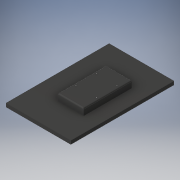
# Autodesk Inventor part: SpectreE165W_16in
Saved by Autodesk Inventor 2019 (Build 230136000, 136)
## iProperties
Created: 2019-05-22
Part Number: SpectreE165W_16in
Material: Generic
Document SubType Name: Modeling
Designer: Jorian Bruslind
Density: 1 g/cm^3
Appearance: Default
Author: Jorian Bruslind
Autodesk Inventor part; units mm, degrees
ref_plane "YZ Plane" through (0, 0, 0) normal (1, 0, 0) x (0, 1, 0)
ref_plane "XZ Plane" through (0, 0, 0) normal (0, 1, 0) x (-1, 0, 0)
ref_plane "XY Plane" through (0, 0, 0) normal (0, 0, 1) x (1, 0, 0)
sketch "Sketch1" plane through (0, 0, 0) normal (0, 1, 0) x (-1, 0, 0)
  line L0 (0, 0) -> (236.22, 0)
  line L1 (236.22, 0) -> (236.22, -375.92)
  line L2 (236.22, -375.92) -> (0, -375.92)
  line L3 (0, -375.92) -> (0, 0)
  dimension "d0" = 236.22
  dimension "d1" = 375.92
  constraints: 8 end point, 2 parallel, 1 horizontal, 1 perpendicular
  measures "d0" distance of L1.end L2.end
  measures "d1" distance of L0.end L1.end
extrude "Extrusion1" add sketch "Sketch1" along normal blind 12.7
sketch "Sketch2" plane through (0, 12.7, 0) normal (0, 1, 0) x (1, 0, 0)
  line L0 (-236.22, 375.92) -> (-236.22, 0) projected
  line L1 (-236.22, 187.96) -> (-147.6375, 187.96)
  line L2 (0, 375.92) -> (-236.22, 375.92) projected
  line L3 (-147.6375, 375.92) -> (-147.6375, 275.92)
  line L4 (-236.22, 0) -> (0, 0) projected
  line L5 (-147.6375, 0) -> (-147.6375, 100)
  line L6 (-147.6375, 0) -> (-47.6375, 0) construction
  line L7 (-147.6375, 275.92) -> (-53.6575, 275.92)
  line L8 (-53.6575, 275.92) -> (-53.6575, 100)
  line L9 (-53.6575, 100) -> (-147.6375, 100)
  line L10 (-147.6375, 100) -> (-147.6375, 275.92)
  dimension "d4" = 88.5825
  dimension "d5" = 100
  dimension "d6" = 88.5825
  dimension "d7" = 100
  dimension "d8" = 90
  dimension "d9" = 88.5825
  dimension "d10" = 93.98
  dimension "d11" = 175.92
  constraints: 16 end point, 3 parallel, 3 perpendicular, 2 horizontal, 2 point on line, 1 midpoint, 1 vertical
  measures "d4" distance of L1.start L1.end
  measures "d5" distance of L3.start L3.end
  measures "d6" distance between parallel lines of L0 L3
  measures "d7" distance of L5.start L5.end
  measures "d8" angle of L6 L5
  measures "d9" distance between parallel lines of L0 L5
  measures "d10" distance of L8.end L9.end
  measures "d11" distance of L7.end L8.end
extrude "Extrusion2" add sketch "Sketch2" along normal blind 25.4 contours L10 L7 L8 L9
fillet "Fillet1" radius 4 4 edges at (-147.6375, 38.1, -187.96) (-53.6575, 38.1, -187.96) (-100.6475, 38.1, -100) (-100.6475, 38.1, -275.92)
sketch "Sketch3" plane through (0, 0, 0) normal (0, -1, 0) x (1, 0, 0)
  line L0 (0, -375.92) -> (0, 0) projected
  line L1 (-236.22, 0) -> (-236.22, -375.92) projected
  line L2 (0, 0) -> (-236.22, -375.92)
  line L3 (-236.22, -375.92) -> (-223.787, -356.1341)
  line L4 (0, 0) -> (-12.433, -19.7859)
  line L5 (-223.787, -356.1341) -> (-12.433, -356.1341)
  line L6 (-12.433, -356.1341) -> (-12.433, -19.7859)
  line L7 (-12.433, -19.7859) -> (-223.787, -19.7859)
  line L8 (-223.787, -19.7859) -> (-223.787, -356.1341)
  dimension "d15" = 23.368
  dimension "d16" = 23.368
  constraints: 14 end point, 2 parallel, 2 point on line, 1 horizontal, 1 perpendicular
  measures "d15" distance of L1.end L3.end
  measures "d16" distance of L0.end L4.end
extrude "Extrusion3" cut sketch "Sketch3" against normal blind 3
sketch "Sketch4" plane through (0, 38.1, 0) normal (0, 1, 0) x (1, 0, 0)
  circle A0 centre (-138.1475, 231.48) radius 1.75
  line L0 (-57.6575, 104) -> (-143.6375, 104) projected
  line L1 (-57.6575, 271.92) -> (-57.6575, 104) projected
  circle A1 centre (-63.1475, 231.48) radius 1.75
  circle A2 centre (-138.1475, 156.48) radius 1.75
  circle A3 centre (-63.1475, 156.48) radius 1.75
  point P0 (0, 0)
  dimension "d19" = 3.5
  dimension "d20" = 127.48
  dimension "d21" = 80.49
  dimension "d24" = 75
  dimension "d27" = 75
  constraints: 4 centre point, 1 horizontal, 1 vertical, 6 other
  measures "d19" diameter of A0
  measures "d20" distance from line of L0 A0.centre
  measures "d21" distance from line of L1 A0.centre
  measures "d24" distance of A0.centre A1.centre
  measures "d27" distance of A0.centre A2.centre
extrude "Extrusion4" cut sketch "Sketch4" against normal blind 3
body "Solid1"
